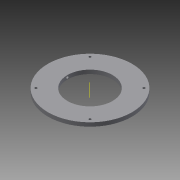
# Autodesk Inventor part: Mirror Support 2
Saved by Autodesk Inventor 2015 (Build 190159000, 159)
## iProperties
Created: 2014-07-17
Part Number: Mirror Support 2
Material: Generic
Document SubType Name: Modeling
Designer: I Rabey
Density: 1 g/cm^3
Appearance: Default
Author: I Rabey
Autodesk Inventor part; units mm, degrees
ref_plane "XZ Plane" through (0, 0, 0) normal (0, 1, 0) x (-1, 0, 0)
ref_plane "XY Plane" through (0, 0, 0) normal (0, 0, 1) x (1, 0, 0)
sketch "Sketch1" plane through (0, 0, 0) normal (0, 1, 0) x (-1, 0, 0)
  circle A0 centre (0, 0) radius 55
  circle A1 centre (0, 0) radius 29.5
  dimension "d0" = 110
  dimension "d1" = 59
  constraints: 2 centre point, 2 coincident
  measures "d0" diameter of A0
  measures "d1" diameter of A1
extrude "Extrusion1" add sketch "Sketch1" along normal blind 5
ref_plane "Work Plane1" through (50, 0, 0) normal (1, 0, 0) x (0, 1, 0)
sketch "Sketch2" plane through (50, 0, 0) normal (1, 0, 0) x (0, 1, 0)
  circle A0 centre (2.5, 0) radius 1.5
  line L0 (5, -55) -> (5, 55) projected
  point P0 (0, 0)
  dimension "d5" = 3
  dimension "d6" = 2.5
  constraints: 1 centre point
  measures "d5" diameter of A0
  measures "d6" distance from line of L0 A0.centre
hole "Hole1" at (50, 2.5, 0) direction (-1, 0, 0) diameter 3 end through all
sketch "Sketch6" plane through (0, 5, 0) normal (0, 1, 0) x (1, 0, 0)
  circle A0 centre (-35.3554, 35.3553) radius 1.5
  circle A1 centre (35.3553, 35.3554) radius 1.5
  circle A2 centre (35.3554, -35.3553) radius 1.5
  circle A3 centre (-35.3553, -35.3554) radius 1.5
  point P0 (0, 0)
  dimension "d30" = 3
  dimension "d31" = 50
  dimension "d32" = 3
  dimension "d33" = 50
  dimension "d34" = 90
  dimension "d35" = 35.3553
  dimension "d36" = 3
  dimension "d37" = 3
  dimension "d38" = 50
  dimension "d39" = 90
  dimension "d40" = 50
  dimension "d41" = 90
  constraints: 4 centre point
  measures "d30" diameter of A0
  measures "d31" distance of point (0, 0) A0.centre
  measures "d32" diameter of A1
  measures "d33" distance of point (0, 0) A1.centre
  measures "d35" vertical distance of point (0, 0) A0.centre
  measures "d36" diameter of A2
  measures "d37" diameter of A3
  measures "d38" distance of A2.centre point (0, 0)
  measures "d40" distance of point (0, 0) A3.centre
extrude "Extrusion6" cut sketch "Sketch6" against normal blind 3
body "Solid1"
